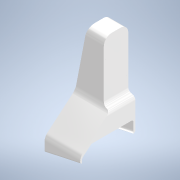
# Autodesk Inventor part: wheelchair_extended_box
Saved by Autodesk Inventor 2021 (Build 250183000, 183)
## iProperties
Created: 2021-05-27
Part Number: wheelchair_extended_box
Material: ABS Plastic
Document SubType Name: Modeling
Designer: Watchdog
Density: 1.06 g/cm^3
Appearance: Smooth - White
Mass: 15746.9 g
Surface Area: 148657 cm^2
Volume: 14855.6 cm^3
Author: Watchdog
Autodesk Inventor part; units mm, degrees
ref_plane "YZ Plane" through (0, 0, 0) normal (1, 0, 0) x (0, 1, 0)
ref_plane "XZ Plane" through (0, 0, 0) normal (0, 1, 0) x (-1, 0, 0)
ref_plane "XY Plane" through (0, 0, 0) normal (0, 0, 1) x (1, 0, 0)
sketch "Sketch1" plane through (0, 0, 0) normal (0, 1, 0) x (-1, 0, 0)
  line L0 (450, -700) -> (-450, -700)
  line L1 (-450, -700) -> (-450, 700)
  line L2 (-450, 700) -> (450, 700)
  line L3 (450, 700) -> (450, -700)
  point P0 (0, 0)
  dimension "d0" = 900
  dimension "d1" = 1400
  dimension "d2" = 700
  dimension "d3" = 450
  constraints: 8 end point, 2 parallel, 1 horizontal, 1 perpendicular
  measures "d0" distance of L0.start L0.end
  measures "d1" distance of L0.end L1.end
  measures "d2" distance from line of point (0, 0) L0
  measures "d3" distance from line of point (0, 0) L3
extrude "Extrusion1" add sketch "Sketch1" along normal blind 1000
sketch "Sketch8" plane through (450, 0, -700) normal (0, 0, -1) x (-1, 0, 0)
  line L0 (900, 1000) -> (0, 1000) projected
  line L1 (180, 1000) -> (180, 2500)
  line L2 (180, 2500) -> (610, 2500)
  line L3 (610, 2500) -> (900, 1000)
  line L4 (0, 0) -> (0, 1000) projected
  point P0 (450, 0)
  dimension "d6" = 1500
  dimension "d7" = 430
  dimension "d8" = 180
  constraints: 6 end point, 1 perpendicular, 1 point on line, 1 vertical
  measures "d6" distance of L1.start L1.end
  measures "d7" distance of L1.end L2.end
  measures "d8" distance between parallel lines of L1 L4
extrude "Extrusion2" add sketch "Sketch8" against normal blind 620
sketch "Sketch9" plane through (-450, 0, -700) normal (-1, 0, 0) x (0, 0, 1)
  line L0 (620, 1000) -> (1400, 1000) projected
  line L1 (620, 1000) -> (1400, 345.5023)
  line L2 (1400, 0) -> (1400, 1000) projected
  point P0 (700, 0)
  dimension "d11" = 40
  constraints: 2 end point, 1 point on line
  measures "d11" angle of L1 L0
extrude "Extrusion3" cut sketch "Sketch9" against normal blind 1000
fillet "Fillet5" radius 100 3 edges at (450, 1000, -390) (270, 1000, -390) (-450, 1000, -390)
fillet "Fillet6" radius 200 4 edges at (0, 345.5023, 700) (-46.8323, 1000, -80) (55, 2500, -80) (55, 2500, -700)
sketch "Sketch16" plane through (0, 0, 0) normal (0, 0, 1) x (1, 0, 0)
  line L0 (-450, 0) -> (-450, 252.2408) projected
  line L1 (-450, 0) -> (650, 233.8122)
  line L2 (650, 233.8122) -> (650, 0)
  line L3 (-450, 0) -> (450, 0) projected
  line L4 (650, 0) -> (-450, 0)
  point P0 (0, 0)
  point P1 (450, 0)
  dimension "d30" = 12
  dimension "d31" = 1100
  constraints: 6 end point, 2 perpendicular
  measures "d30" angle of L3 L1
  measures "d31" distance from line of L0.start L2
extrude "Extrusion7" cut sketch "Sketch16" along normal mid plane 1500
fillet "Fillet7" radius 50 2 edges at (0, 95.6505, -700) (0, 95.6505, 700)
shell "Shell2" thickness 2 removed faces 0
sketch "Sketch18" plane through (0, 0, 0) normal (0, 1, 0) x (-1, 0, 0)
  line L0 (444, -650) -> (-799.8657, -650)
  line L1 (-799.8657, -650) -> (-799.8657, 650)
  line L2 (-799.8657, 650) -> (444, 650)
  line L3 (444, 650) -> (444, -650)
  line L4 (-450, 700) -> (450, 700) projected
  line L5 (450, -700) -> (-450, -700) projected
  line L6 (450, -650) -> (450, 650) projected
  point P0 (0, 0)
  dimension "d39" = 50
  dimension "d40" = 50
  dimension "d41" = 6
  constraints: 8 end point, 2 parallel, 1 horizontal, 1 perpendicular
  measures "d39" distance between parallel lines of L4 L2
  measures "d40" distance between parallel lines of L5 L0
  measures "d41" distance between parallel lines of L6 L3
extrude "Extrusion8" cut sketch "Sketch18" along normal blind 300
sketch "Sketch19" plane through (450, 900, 39.1754) normal (1, 0, 0) x (0, 0, -1)
  line L0 (689.1754, -600) -> (-610.8246, -600) projected
  line L1 (689.1754, -600) -> (689.1754, -400)
  line L2 (689.1754, -400) -> (-372.4739, -400)
  line L3 (-372.4739, -400) -> (-610.8246, -600)
  line L4 (0, 0) -> (-589.3822, -494.5504) projected
  point P0 (39.1754, -900)
  dimension "d44" = 200
  constraints: 6 end point, 1 parallel, 1 perpendicular, 1 vertical
  measures "d44" distance between parallel lines of L0 L2
extrude "Extrusion9" cut sketch "Sketch19" against normal blind 300
fillet "Fillet8" radius 50 3 edges at (449, 500, -650) (449, 500, 411.6493) (449, 300, 650)
sketch "Sketch20" plane through (-196.6296, 2300, -698) normal (0, 0, 1) x (1, 0, 0)
  line L0 (-253.3704, -2248.883) -> (-253.3704, -1309.578) projected
  point P0 (196.6296, -2300)
  point P1 (-43.3704, -1788.883)
  dimension "d48" = 210
  dimension "d49" = 460
  measures "d48" distance from line of L0 point (-43.37, -1788.883)
  measures "d49" vertical distance of L0.start point (-43.37, -1788.883)
hole "Hole1" at (-240, 511.117, -698) direction (0, 0, -1) diameter 10 end through all
sketch "Sketch21" plane through (270, 1098.9975, -80) normal (1, 0, 0) x (0, 0, -1)
  circle A0 centre (565.1575, 277.2473) radius 5
  circle A1 centre (40, 903.1057) radius 5
  circle A2 centre (445.4299, 1243.3017) radius 5
  line L0 (575.5881, 1352.5174) -> (0, 869.5417)
  line L1 (620, 0) -> (0, 0) projected
  line L2 (0, 0) -> (0, 1201.0025) projected
  line L3 (620, 1201.0025) -> (620, 0) projected
  line L4 (40, 903.1057) -> (565.1575, 277.2473)
  line L5 (40, 903.1057) -> (0, 950.7758)
  line L6 (0, 1201.0025) -> (0, -5.736) projected
  point P0 (-80, -1098.9975)
  dimension "d57" = 40
  dimension "d64" = 10
  dimension "d65" = 10
  dimension "d66" = 10
  dimension "d71" = 817
  dimension "d75" = 40
  constraints: 8 end point, 4 point on line, 3 centre point, 2 perpendicular
  measures "d57" angle of L1 L0
  measures "d64" diameter of A2
  measures "d65" diameter of A1
  measures "d66" diameter of A0
  measures "d71" distance of L4.start L4.end
  measures "d75" distance from line of L2 L4.start
extrude "Extrusion10" cut sketch "Sketch21" against normal blind 12 contours A0 | A1 L4 L0 | L0 L5 A1 | A1 L0 L4 | L5 L0 A1 | A2 L0 | L0 A2
sketch "Sketch22" plane through (-450, 990.422, -700) normal (-1, 0, 0) x (0, 0, 1)
  line L0 (-43.9778, -850.6351) -> (145.4226, -1009.561)
  line L1 (-53.3391, -1089.9912) -> (-43.9778, -850.6351)
  line L2 (-53.3391, -1089.9912) -> (87.3459, -1089.9912)
  line L3 (87.3459, -1089.9912) -> (145.4226, -1009.561)
  line L4 (1328.5575, -584.9724) -> (691.4425, -50.3694) projected
  point P0 (700, -990.422)
  point P1 (-44.1322, -854.5823)
  constraints: 8 end point, 1 horizontal, 1 parallel
extrude "Extrusion11" cut sketch "Sketch22" against normal blind 400
sketch "Sketch24" plane through (-450, 102.8851, -700) normal (0, -0.7660444, -0.6427876) x (1, 0, 0)
  ellipse E0 centre (46.1671, 65.2704) end of major axis (357.2105, 22.7729) minor radius 50 (243.5498, 0) -> (286.6539, 65.2704) ccw projected
  line L0 (286.6539, 65.2704) -> (0, 180.788)
  line L1 (0, 160.0609) -> (0, 1100.2933) projected
  line L2 (0, 0) -> (243.5498, 0)
  line L3 (0, 180.788) -> (0, 0)
  line L4 (6, 158.0768) -> (6, 1099.4735) projected
  point P0 (450, 602.3644)
  constraints: 6 end point, 1 horizontal, 1 parallel, 1 point on line, 2 other
extrude "Extrusion13" add sketch "Sketch24" along normal blind 2
equation "\"d2\" = 0.5 * d1"
equation "\"d3\" = 0.5 * d0"
equation "\"d65\" = d64"
equation "\"hoop_angle_z\" = 45deg"
equation "\"hoop_bearing_length\" = 5deg"
equation "\"hoop_cable_diam\" = 5"
equation "\"hoop_cable_pulley_diam\" = 22"
equation "\"hoop_thickness_large\" = 4"
equation "\"hoop_thickness_medium\" = 3.2"
equation "\"hoop_thickness_small\" = 2"
equation "\"hoop_width_large\" = 51"
equation "\"hoop_width_medium\" = 33.7"
equation "\"hoop_width_small\" = 25.4"
equation "\"rack_tooth_addendum\" = 5"
equation "\"rack_tooth_dedendum\" = 5"
equation "\"rack_tooth_thickness\" = 5"
equation "\"secure_arm_angle\" = 35deg"
equation "\"secure_arm_radii\" = 9"
equation "\"support_baseClamp_platformLengthBuffer\" = 35"
equation "\"support_baseClamp_platformThickness\" = 15"
equation "\"support_baseClamp_platformWidthBuffer\" = 0"
equation "\"support_baseClamp_sleeveHoleDiameter\" = 12"
equation "\"support_baseClamp_sleeveSweepTerminationAngle\" = 55deg"
equation "\"support_baseClamp_thickness\" = 8"
equation "\"support_frame_endHoleBuffer\" = 45"
equation "\"support_frame_squareBarFillet\" = 2"
equation "\"support_frame_squareBarThickness\" = 5"
equation "\"hoop_tabs_thickness\" = 6"
equation "\"hoop_tabs_hole\" = 12"
equation "\"wheelchair_deployed_width\" = 635"
equation "\"wheelchair_deployed_length\" = 1067"
equation "\"wheelchair_deployed_height\" = 914"
equation "\"sm_varx_member_tolerance\" = 0"
equation "\"sm_varx_pinPlate_holeDiameter\" = 5"
equation "\"sm_varx_pinPlate_thickness\" = 5"
equation "\"sm_varx_squareBarThickness\" = 2.5"
equation "\"hoop_bushing23_radialInterference\" = 0"
equation "\"hoop_bushing12_radialInterference\" = 0"
equation "\"hoop_bushing12_od\" = -2 * hoop_thickness_large + hoop_width_large + hoop_bushing12_radialInterference"
equation "\"hoop_bushing23_od\" = -2 * hoop_thickness_medium + hoop_width_medium + hoop_bushing23_radialInterference"
equation "\"wheelchatir_pos_deploy_angle_0\" = 65deg"
equation "\"wheelchatir_pos_store_angle_0\" = 90deg"
equation "\"wheelchatir_pos_deploy_angle_1\" = 20deg"
equation "\"wheelchatir_pos_store_angle_1\" = 20deg"
equation "\"hoop_bushing12_thickness\" = -hoop_width_medium + hoop_bushing12_od - 2 * hoop_bushing12_radialInterference"
equation "\"hoop_bushing23_thickness\" = -hoop_width_small + hoop_bushing23_od - 2 * hoop_bushing23_radialInterference"
body "Solid1"
